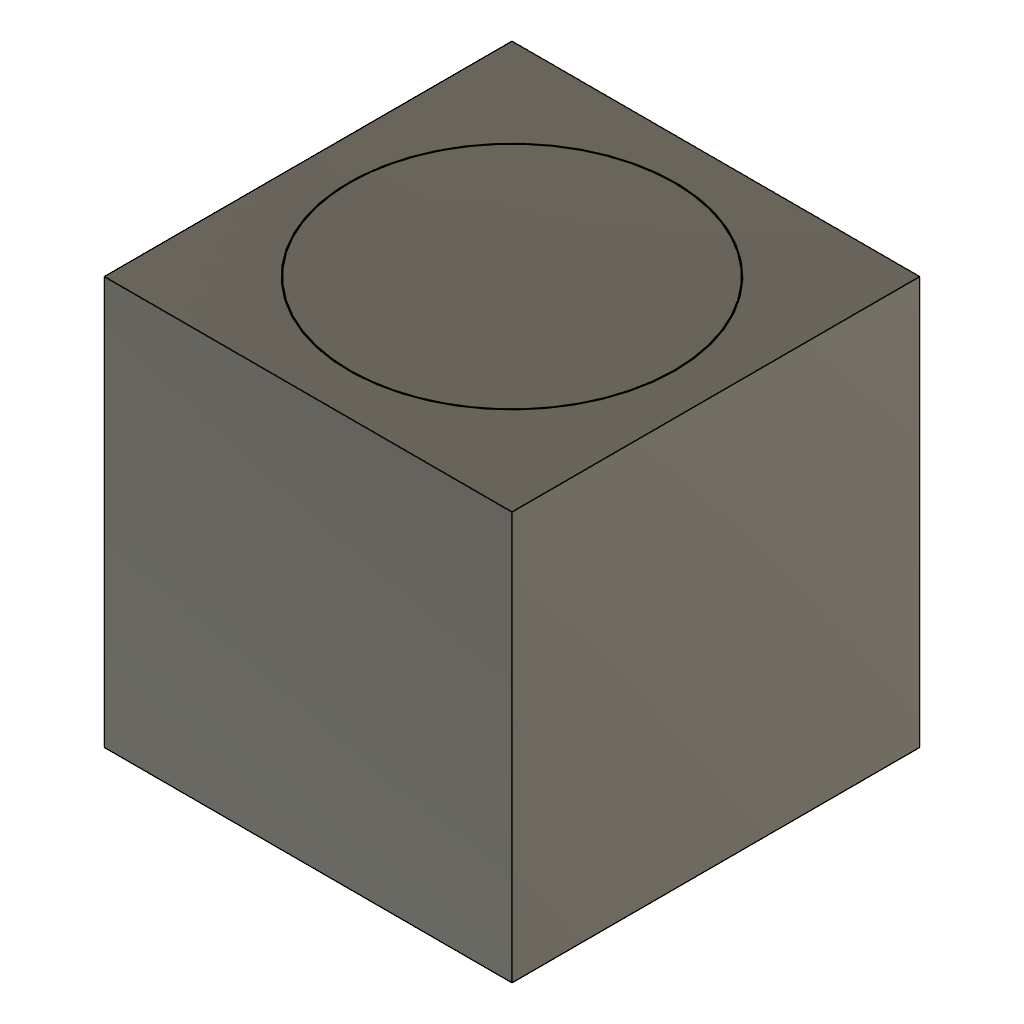
cube-tolerance-v1 (Autodesk Fusion 360 design; units mm, degrees)
part number: 2026-09-11-17-29-46-284
Autodesk Fusion 360 part; units mm, degrees
sketch "Sketch3" plane through (0, 0, 0) normal (0, 1, 0) x (1, 0, 0)
  line L0 (25, -25) -> (-25, -25)
  line L1 (-25, -25) -> (-25, 25)
  line L2 (-25, 25) -> (25, 25)
  line L3 (25, 25) -> (25, -25)
  line L4 (25, -25) -> (-25, 25) construction
  line L5 (-25, -25) -> (25, 25) construction
  dimension "d1" = 50
  dimension "d2" = 50
  constraint horizontal L0
  constraint perpendicular L0 L1
  constraint parallel L0 L2
  constraint parallel L1 L3
  constraint coincident L4 origin
  constraint coincident L5 origin
  measures "d1" distance of L1.end L2.end
  measures "d2" distance of L0.end L1.end
extrude "Extrude1" add sketch "Sketch3" along normal blind 50 makes body 1
sketch "Sketch4" plane through (0, 0, 25) normal (0, 0, 1) x (-1, 0, 0)
  line L0 (25, 0) -> (-25, 0)
  line L1 (-25, 0) -> (-25, -50)
  line L2 (-25, -50) -> (25, -50)
  line L3 (25, -50) -> (25, 0)
  circle A0 centre (0, -25) radius 20
  dimension "d5" = 40
  measures "d5" diameter of A0
extrude "Extrude2" cut sketch "Sketch4" against normal blind 75 contours A0 bodies 1
sketch "Sketch5" plane through (0, 0, 25) normal (0, 0, 1) x (-1, 0, 0)
  circle A0 centre (0, -25) radius 20
  line L0 (25, 0) -> (-25, 0)
  line L1 (-25, 0) -> (-25, -50)
  line L2 (-25, -50) -> (25, -50)
  line L3 (25, -50) -> (25, 0)
  circle A1 centre (0, -25) radius 19.9
  dimension "d9" = 39.8
  constraint concentric A0 A1
  measures "d9" diameter of A1
extrude "Extrude3" add sketch "Sketch5" against normal blind 50 separate body contours A1 makes body 2
equation "gap = 0.2 mm"
equation "d9 = 40 mm - gap"
